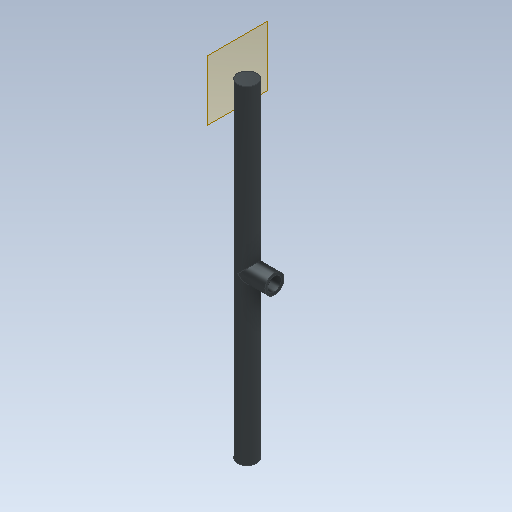
# Autodesk Inventor part: trail 5
Saved by Autodesk Inventor 2020.2 (Build 242310000, 310)
## iProperties
Created: 2020-02-13
Part Number: trail 5
Material: Iron, Cast
Document SubType Name: Modeling
Designer: lenovo
Density: 7.15 g/cm^3
Appearance: Iron Gray
Author: lenovo
Autodesk Inventor part; units mm, degrees
ref_plane "YZ Plane" through (0, 0, 0) normal (1, 0, 0) x (0, 1, 0)
ref_plane "XZ Plane" through (0, 0, 0) normal (0, 1, 0) x (-1, 0, 0)
ref_plane "XY Plane" through (0, 0, 0) normal (0, 0, 1) x (1, 0, 0)
sketch "Sketch1" plane through (0, 0, 0) normal (0, 1, 0) x (-1, 0, 0)
  point P0 (0, 0)
sketch "Sketch2" plane through (0, 0, 0) normal (0, 1, 0) x (-1, 0, 0)
  circle A0 centre (0, 0) radius 2.5
  circle A1 centre (0, 0) radius 3.5
  dimension "d0" = 5
  dimension "d1" = 7
  constraints: 2 centre point, 2 coincident
  measures "d0" diameter of A0
  measures "d1" diameter of A1
extrude "Extrusion1" add sketch "Sketch2" along normal blind 110
sketch "Sketch3" plane through (0, 110, 0) normal (0, 1, 0) x (1, 0, 0)
  circle A0 centre (0, 0) radius 3.5
  constraints: 1 centre point, 1 coincident
extrude "Extrusion2" add sketch "Sketch3" along normal blind 5
sketch "Sketch4" plane through (0, 0, 0) normal (0, -1, 0) x (1, 0, 0)
  circle A0 centre (0, 0) radius 3.5
  constraints: 1 centre point, 1 coincident
extrude "Extrusion3" add sketch "Sketch4" along normal blind 5
sketch "Sketch5" plane through (0, 0, 0) normal (0, 0, 1) x (1, 0, 0)
  point P0 (0, 0)
sketch "Sketch6" plane through (0, 0, 0) normal (1, 0, 0) x (0, 1, 0)
  circle A0 centre (55, 0) radius 2.5
  circle A1 centre (55, 0) radius 3.5
  point P0 (0, 0)
  dimension "d8" = 5
  dimension "d9" = 7
  constraints: 2 centre point, 1 coincident
  measures "d8" diameter of A0
  measures "d9" diameter of A1
extrude "Extrusion4" add sketch "Sketch6" along normal blind 10
sketch "Sketch7" plane through (0, 0, 0) normal (0, 0, 1) x (1, 0, 0)
  line L0 (-3.5, -5) -> (3.5, -5) projected
  line L1 (-3.5, -5) -> (-3.5, 115)
  line L2 (-3.5, -5) -> (-3.5, 115) projected
  point P0 (0, 0)
  constraints: 2 end point, 1 point on line
ref_plane "Work Plane5" through (-3.5, 115, 0) normal (1, 0, 0) x (0, 1, 0)
sketch "Sketch8" plane through (-3.5, 115, 0) normal (1, 0, 0) x (0, 1, 0)
  circle A0 centre (-10, 0) radius 0.5
  circle A1 centre (-20, 0) radius 0.5
  circle A2 centre (-30, 0) radius 0.5
  circle A3 centre (-40, 0) radius 0.5
  circle A4 centre (-50, 0) radius 0.5
  point P0 (-115, 0)
  dimension "d12" = 1
  dimension "d13" = 1
  dimension "d14" = 1
  dimension "d15" = 1
  dimension "d16" = 1
  constraints: 5 centre point
  measures "d12" diameter of A0
  measures "d13" diameter of A1
  measures "d14" diameter of A2
  measures "d15" diameter of A3
  measures "d16" diameter of A4
extrude "Extrusion5" cut sketch "Sketch8" against normal mid plane 3
ref_plane "Work Plane7" through (-3.5, 115, 0) normal (1, 0, 0) x (0, 1, 0)
sketch "Sketch9" plane through (-3.5, 115, 0) normal (1, 0, 0) x (0, 1, 0)
  circle A0 centre (-60, 0) radius 0.5
  circle A1 centre (-70, 0) radius 0.5
  circle A2 centre (-80, 0) radius 0.5
  circle A3 centre (-90, 0) radius 0.5
  circle A4 centre (-100, 0) radius 0.5
  circle A5 centre (-110, 0) radius 0.5
  point P0 (-115, 0)
  dimension "d19" = 1
  dimension "d20" = 1
  dimension "d21" = 1
  dimension "d22" = 1
  dimension "d23" = 1
  dimension "d24" = 1
  constraints: 6 centre point
  measures "d19" diameter of A0
  measures "d20" diameter of A1
  measures "d21" diameter of A2
  measures "d22" diameter of A3
  measures "d23" diameter of A4
  measures "d24" diameter of A5
extrude "Extrusion6" cut sketch "Sketch9" along normal mid plane 3 contours A1 | A2 | A3 | A4 | A5
body "Solid1"
